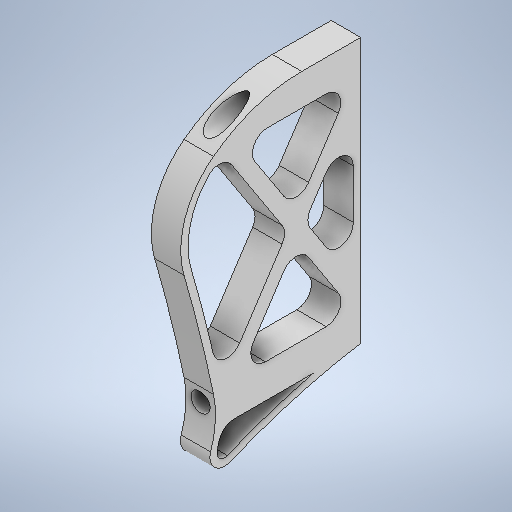
# Autodesk Inventor part: Harp Ring Pusher
Saved by Autodesk Inventor 2025.1 (Build 291241020, 241B)
## iProperties
Created: 2024-12-11
Part Number: Harp Ring Pusher
Material: Generic
Document SubType Name: Modeling
Designer: AtuStem
Mass: 49.5398 g
Surface Area: 261.99 cm^2
Volume: 49.5398 cm^3
Density: 1 g/cm^3
Appearance: Default
Author: AtuStem
## iProperties of the stored document Harp Ring Pusher_3DPrint.ipt
Created: 2024-12-11
Part Number: Harp Ring Pusher_3DPrint
Material: Generic
Document SubType Name: Modeling
Designer: AtuStem
Density: 1 g/cm^3
Appearance: Default
Author: AtuStem
Autodesk Inventor part; units mm, degrees
ref_plane "YZ Plane" through (0, 0, 0) normal (1, 0, 0) x (0, 1, 0)
ref_plane "XZ Plane" through (0, 0, 0) normal (0, 1, 0) x (-1, 0, 0)
ref_plane "XY Plane" through (0, 0, 0) normal (0, 0, 1) x (1, 0, 0)
sketch "Sketch1" plane through (0, 0, 0) normal (1, 0, 0) x (0, 1, 0)
  line L0 (0, 0) -> (0, 76.2) construction
  line L1 (38.1, 0) -> (38.1, 63.5) construction
  line L2 (-50.8, 0) -> (-50.8, 63.5) construction
  line L3 (-50.8, 91.6102) -> (-12.7, 91.6102) construction
  line L4 (-88.9, 0) -> (-88.9, 76.2) construction
  line L5 (50.8, 0) -> (50.8, 25.4)
  arc A0 (50.8, 25.4) -> (38.1, 63.5) centre (-12.7, 25.4) ccw
  arc A1 (38.1, 63.5) -> (0, 76.2) centre (9.8778, 42.3333) ccw
  line L6 (50.8, 0) -> (-88.9, 0)
  arc A2 (-50.8, 63.5) -> (0, 76.2) centre (-188.9125, 723.9) ccw
  arc A3 (-88.9, 76.2) -> (-50.8, 63.5) centre (-58.9603, 102.5192) ccw
  arc A4 (-63.5, 0) -> (-88.9, 76.2) centre (-314.1344, -41.2115) ccw
  dimension "d1" = 76.2
  dimension "d3" = 63.5
  dimension "d4" = 38.1
  dimension "d5" = 63.5
  dimension "d7" = 50.8
  dimension "d10" = 76.2
  dimension "d11" = 38.1
  dimension "d12" = 25.4
  dimension "d13" = 12.7
  dimension "d14" = 12.7
  dimension "d15" = 254
  constraints: 14 end point, 10 point on circle, 5 centre point, 5 vertical, 4 tangent, 2 horizontal, 1 point on line
  measures "d1" distance of L0.start L0.end
  measures "d3" distance of L1.start L1.end
  measures "d4" distance between parallel lines of L0 L1
  measures "d5" distance of L2.start L2.end
  measures "d7" distance between parallel lines of L2 L0
  measures "d10" distance of L4.start L4.end
  measures "d11" distance between parallel lines of L4 L2
  measures "d12" distance of L5.start L5.end
  measures "d13" distance between parallel lines of L1 L5
  measures "d14" distance from line of L2 A4.start
  measures "d15" radius of A4
extrude "Extrusion1" add sketch "Sketch1" along normal blind 12.7
ref_plane "Work Plane1" through (0, 9.8778, 77.6111) normal (0, 0, -1) x (-1, 0, 0)
sketch "Sketch2" plane through (0, 9.8778, 77.6111) normal (0, 0, -1) x (-1, 0, 0)
  line L0 (0, -73.3778) -> (0, 40.9222) construction
  line L1 (0, 40.9222) -> (-12.7, 40.9222) construction
  line L2 (-12.7, -73.3778) -> (-12.7, 40.9222) construction
  line L3 (0, -73.3778) -> (-12.7, -73.3778) construction
  line L4 (-6.35, 40.9222) -> (-6.35, 34.5722) construction
  line L5 (0, 28.2222) -> (-12.7, 28.2222) projected
  line L6 (-6.35, 34.5722) -> (-6.35, -67.0278) construction
  point P0 (0, -9.8778)
  dimension "d18" = 6.35
  dimension "d20" = 101.6
  constraints: 4 end point, 2 coincident, 1 midpoint, 1 perpendicular, 1 vertical
  measures "d18" distance of L4.start L4.end
  measures "d20" distance of L4.end L6.end
sketch3d "3D Sketch1"
hole "Hole1" at (6.35, 44.45, 53.079) direction (0, 0, -1) diameter 4.6482 end through all start extended yes counterbore diameter 8.255 counterbore depth 40.386
hole "Hole2" at (6.35, -57.15, 62.697) direction (0, 0, -1) diameter 4.6482 end through all start extended yes counterbore diameter 8.255 counterbore depth 49.9872
fillet "Fillet1" radius 6.35 1 edges at (6.35, -88.9, 76.2)
sketch "Sketch3" plane through (0, 0, 0) normal (-1, 0, 0) x (0, 0, 1)
  line L0 (12.693, 40.3225) -> (12.693, 48.5775) construction
  line L1 (12.7098, -61.2775) -> (12.7098, -53.0225) construction
  line L2 (0, 37.1475) -> (3.175, 37.1475)
  arc A0 (56.2923, -79.5944) -> (64.7468, -71.7013) centre (58.7299, -73.7309) ccw projected
  arc A1 (63.5, -50.8) -> (64.7468, -71.7013) centre (102.5192, -58.9603) ccw projected
  arc A2 (76.2, 0) -> (63.5, -50.8) centre (723.9, -188.9125) ccw projected
  arc A3 (76.2, 0) -> (63.5, 38.1) centre (42.3333, 9.8778) ccw projected
  arc A4 (63.5, 38.1) -> (25.4, 50.8) centre (25.4, -12.7) ccw projected
  line L3 (0, 50.8) -> (25.4, 50.8) projected
  line L4 (0, -63.5) -> (0, 50.8) projected
  arc A5 (56.2923, -79.5944) -> (0, -63.5) centre (-41.2115, -314.1344) ccw projected
  line L5 (0, -49.8475) -> (3.175, -49.8475)
  line L6 (69.357, -25.2767) -> (66.2768, -24.5067)
  line L7 (75.8008, 21.0336) -> (72.7887, 20.0296)
  line L8 (12.7098, -61.2775) -> (62.7232, -61.2775) projected
  line L9 (63.0633, -78.3725) -> (60.8966, -76.0517)
  line L10 (12.7098, -53.0225) -> (63.1005, -53.0225) projected
  line L11 (37.9051, -53.0225) -> (37.9051, -49.8475)
  line L12 (3.175, 37.1475) -> (3.175, -49.8475)
  line L13 (64.1848, 37.5732) -> (62.2181, 35.0806)
  arc A6 (72.7887, 20.0296) -> (62.2181, 35.0806) centre (42.3333, 9.8778) ccw
  line L14 (76.2, 0) -> (73.152, 0.889)
  arc A7 (73.152, 0.889) -> (72.7887, 20.0296) centre (42.3333, 9.8778) ccw
  line L15 (3.175, 37.1475) -> (59.5985, 37.1475) construction
  line L16 (62.2181, 35.0806) -> (59.5985, 37.1475)
  line L17 (3.175, 37.1475) -> (59.5985, 37.1475)
  arc A8 (73.152, 0.889) -> (66.2768, -24.5067) centre (723.9, -188.9125) ccw
  line L18 (63.6999, -49.8475) -> (60.5931, -49.1931)
  arc A9 (66.2768, -24.5067) -> (60.5931, -49.1931) centre (723.9, -188.9125) ccw
  line L19 (3.175, -49.8475) -> (60.4552, -49.8475)
  line L20 (60.5931, -49.1931) -> (60.4552, -49.8475)
  circle A10 centre (58.7299, -73.7309) radius 3.175
  line L21 (58.7575, -61.2775) -> (58.7575, -64.4525)
  line L22 (63.4849, -67.0479) -> (60.3759, -67.692)
  line L23 (20.4158, -61.2775) -> (20.4158, -64.4525)
  line L24 (20.4158, -64.4525) -> (19.6549, -67.535)
  arc A11 (57.5111, -76.6627) -> (20.4158, -64.4525) centre (-41.2115, -314.1344) ccw
  arc A12 (56.2923, -79.5944) -> (0, -63.5) centre (-41.2115, -314.1344) ccw projected
  line L25 (20.4158, -64.4525) -> (58.7575, -64.4525)
  arc A13 (58.7575, -64.4525) -> (60.3759, -67.692) centre (248.1884, 28.1605) ccw
  arc A14 (61.9033, -73.6307) -> (60.3759, -67.692) centre (47.8711, -74.074) ccw
  point P0 (0, 0)
  point P1 (60.3409, 40.3225)
  dimension "d44" = 3.175
  dimension "d45" = 3.175
  dimension "d48" = 3.175
  dimension "d49" = 3.175
  dimension "d50" = 3.175
  dimension "d51" = 3.175
  dimension "d53" = 3.175
  dimension "d54" = 3.175
  dimension "d55" = 3.175
  dimension "d56" = 3.175
  dimension "d58" = 3.175
  dimension "d60" = 3.175
  dimension "d61" = 3.175
  dimension "d62" = 3.175
  constraints: 40 end point, 24 point on circle, 8 centre point, 8 line through centre, 7 tangent, 4 horizontal, 4 vertical, 3 point on line, 1 coincident, 1 collinear, 1 concentric, 1 equal length, 1 midpoint
  measures "d44" distance of L2.start L2.end
  measures "d45" distance from line of L2 L0.start
  measures "d48" distance of L5.start L5.end
  measures "d49" distance from line of L1.end L5
  measures "d50" distance of L6.start L6.end
  measures "d51" distance of L7.start L7.end
  measures "d53" distance of L9.start L9.end
  measures "d54" distance of L11.start L11.end
  measures "d55" distance of L13.start L13.end
  measures "d56" distance of L14.start L14.end
  measures "d58" distance of L18.start L18.end
  measures "d60" distance of L21.start L21.end
  measures "d61" distance of L22.start L22.end
  measures "d62" distance of L23.start L23.end
extrude "Extrusion2" cut sketch "Sketch3" against normal blind 15.24 contours L17 L16 A6 A7 A8 A9 L20 L19 L12 | L25 A13 A14 A10 A11 | A10
sketch "Sketch4" plane through (12.7, 0, 0) normal (1, 0, 0) x (0, 0, -1)
  line L0 (-59.5985, 37.1475) -> (-3.175, 37.1475) projected
  line L1 (-62.2181, 35.0806) -> (-59.5985, 37.1475) projected
  arc A0 (-62.2181, 35.0806) -> (-73.152, 0.889) centre (-42.3333, 9.8778) ccw projected
  arc A1 (-60.5931, -49.1931) -> (-73.152, 0.889) centre (-723.9, -188.9125) ccw projected
  line L2 (-3.175, -49.8475) -> (-60.4552, -49.8475) projected
  line L3 (-60.4552, -49.8475) -> (-60.5931, -49.1931) projected
  line L4 (-3.175, 37.1475) -> (-3.175, -49.8475) projected
  line L5 (-52.0298, 37.1475) -> (-27.7865, -0.2314)
  line L6 (-24.0137, -6.0484) -> (-3.175, -38.178)
  line L7 (-59.5985, 37.1475) -> (-31.5993, -6.0222)
  line L8 (-27.8265, -11.8392) -> (-3.175, -49.8475)
  line L9 (-60.4552, -49.8475) -> (-31.5993, -6.0222)
  line L10 (-27.7865, -0.2314) -> (-3.175, 37.1475)
  line L11 (-52.8524, -49.8475) -> (-27.8265, -11.8392)
  line L12 (-24.0137, -6.0484) -> (-3.175, 25.6006)
  point P0 (0, 0)
  constraints: 16 end point, 8 parallel, 4 point on line
extrude "Extrusion3" add sketch "Sketch4" against normal up to surface (12.7 mm away) contours L0 L5 L10 L4 L12 L6 L8 L11 L2 L9 L7
fillet "Fillet2" radius 6.35 12 edges at (6.35, 37.1475, 52.0298) (6.35, -0.2314, 27.7865) (6.35, 37.1475, 3.175) (6.35, 25.6006, 3.175) (6.35, -6.0484, 24.0137) (6.35, -38.178, 3.175) (6.35, -6.0222, 31.5993) (6.35, -11.8392, 27.8265) (6.35, -49.8475, 52.8524) (6.35, -49.8475, 3.175) (6.35, 37.1475, 59.5985) (6.35, -49.8475, 60.4552)
fillet "Fillet3" radius 6.35 1 edges at (6.35, -64.4525, 58.7575)
body "Solid1"
